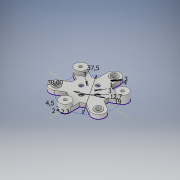
# Autodesk Inventor part: PlanetaryHolderTop
Saved by Autodesk Inventor 2018.3 (Build 223284000, 284)
## iProperties
Created: 2018-07-08
Part Number: PlanetaryHolderTop
Material: Generisch
Document SubType Name: Modeling
Designer: JochenAlt
Density: 1 g/cm^3
Appearance: Vorgabe
Author: JochenAlt
Autodesk Inventor part; units mm, degrees
note: some values were not read from the file. Chosen so that the rebuilt part matches the saved one: sketch regions of "Extrusion1".
ref_plane "YZ Plane" through (0, 0, 0) normal (1, 0, 0) x (0, 1, 0)
ref_plane "XZ Plane" through (0, 0, 0) normal (0, 1, 0) x (-1, 0, 0)
ref_plane "XY Plane" through (0, 0, 0) normal (0, 0, 1) x (1, 0, 0)
sketch "Skizze1" plane through (0, 0, 0) normal (0, 0, 1) x (1, 0, 0)
  circle A0 centre (0, 0) radius 18.75 construction
  circle A1 centre (0, 0) radius 9.5
  circle A2 centre (0, 18.75) radius 2
  line L0 (0, 0) -> (-16.238, -9.375) construction
  line L1 (0, 33.1) -> (0, -32.35) construction
  line L2 (-32.2953, 0) -> (32.2953, 0) construction
  circle A3 centre (0, 0) radius 6.35 construction
  circle A4 centre (0, 6.35) radius 1.5
  circle A5 centre (0, -6.35) radius 1.5
  circle A6 centre (6.35, 0) radius 1.5
  circle A7 centre (-6.35, 0) radius 1.5
  arc A8 (-5, 11.4564) -> (5, 11.4564) centre (0, 0) ccw
  arc A9 (5, 18.75) -> (-5, 18.75) centre (0, 18.75) ccw
  line L3 (-5, 18.75) -> (-5, 11.4564)
  line L4 (5, 18.75) -> (5, 11.4564)
  circle A10 centre (16.238, -9.375) radius 2
  arc A11 (13.738, -13.7051) -> (18.738, -5.0449) centre (16.238, -9.375) ccw
  line L5 (18.738, -5.0449) -> (12.4216, -1.3981)
  line L6 (13.738, -13.7051) -> (7.4216, -10.0583)
  circle A12 centre (-16.238, -9.375) radius 2
  arc A13 (-18.738, -5.0449) -> (-13.738, -13.7051) centre (-16.238, -9.375) ccw
  line L7 (-18.738, -5.0449) -> (-12.4216, -1.3981)
  line L8 (-13.738, -13.7051) -> (-7.4216, -10.0583)
  circle A14 centre (0, 18.75) radius 3
  circle A15 centre (16.238, -9.375) radius 3
  circle A16 centre (-16.238, -9.375) radius 3
  circle A17 centre (0, -18.75) radius 1.15
  circle A18 centre (16.238, 9.375) radius 1.15
  circle A19 centre (-16.238, 9.375) radius 1.15
  circle A20 centre (16.238, 9.375) radius 2.25
  circle A21 centre (0, -18.75) radius 2.25
  circle A22 centre (-16.238, 9.375) radius 2.25
  arc A23 (18.363, 5.6944) -> (14.113, 13.0556) centre (16.238, 9.375) ccw
  arc A24 (-4.25, -18.75) -> (4.25, -18.75) centre (0, -18.75) ccw
  arc A25 (-14.113, 13.0556) -> (-18.363, 5.6944) centre (-16.238, 9.375) ccw
  line L9 (18.363, 5.6944) -> (12.3054, 2.1971)
  line L10 (14.113, 13.0556) -> (8.0554, 9.5583)
  line L11 (4.25, -11.7553) -> (4.25, -18.75)
  line L12 (-4.25, -11.7553) -> (-4.25, -18.75)
  line L13 (-8.0554, 9.5583) -> (-14.113, 13.0556)
  line L14 (-12.3054, 2.1971) -> (-18.363, 5.6944)
  circle A26 centre (0, -18.75) radius 4.25
  circle A27 centre (16.238, 9.375) radius 4.25
  circle A28 centre (-16.238, 9.375) radius 4.25
  dimension "d0" = 37.5
  dimension "d1" = 4
  dimension "d2" = 30
  dimension "d3" = 19
  dimension "d4" = 12.7
  dimension "d5" = 3
  dimension "d7" = 3
  dimension "d8" = 3
  dimension "d17" = 1
  dimension "d20" = 2.3
  dimension "d22" = 2
  dimension "d23" = 4.5
  constraints: 28 centre point, 26 end point, 23 point on circle, 21 coincident, 17 equal radius, 12 tangent, 7 point on line, 4 parallel, 2 vertical, 22 other
  measures "d0" diameter of A0
  measures "d1" diameter of A2
  measures "d2" angle of L0 L2
  measures "d3" diameter of A1
  measures "d4" diameter of A3
  measures "d5" diameter of A4
  measures "d8" radial gap between concentric circles of A2 A9
  measures "d17" radial gap between concentric circles of A14 A2
  measures "d20" diameter of A17
  measures "d22" radial gap between concentric circles of A24 A21
  measures "d23" diameter of A21
extrude "Extrusion1" add sketch "Skizze1" along normal blind 3 contours A1 | A2 | L3 A9 L4 A8 | A8 L14 A28 L13 | A28 A25 | A8 L8 A13 L7 | L10 A27 L9 A8 | A8 L11 A26 L12 | A23 A27 | A26 A24 | L5 A11 L6 A8 | A10 | A12 | A14 | A15 | A16
extrude "Extrusion3" cut sketch "Skizze1" along normal blind 2 contours A1
extrude "Extrusion4" cut sketch "Skizze1" against normal blind 2 from surface at 3 contours A2 | A10 | A12
extrude "Extrusion5" add sketch "Skizze1" along normal blind 0.5 from surface at 3 contours A14 | A15 | A16
extrude "Extrusion6" add sketch "Skizze1" along normal blind 3 from surface at 3 contours A28 A25 | A23 A27 | A26 A24 | A20 | A21 | A22
